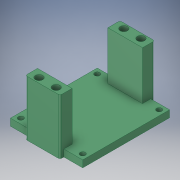
# Autodesk Inventor part: МД.001.1000 - Опора захвата
Saved by Autodesk Inventor 2019 (Build 230136000, 136)
## iProperties
Created: 2019-12-30
Part Number: МД.001.1000 - Опора захвата
Material: Пластик АБС
Document SubType Name: Modeling
Designer: Петров Иван
Density: 1.06 g/cm^3
Appearance: Гладкий — темный цвет морской волны
Author: Петров Иван
Autodesk Inventor part; units mm, degrees
ref_plane "YZ Plane" through (0, 0, 0) normal (1, 0, 0) x (0, 1, 0)
ref_plane "XZ Plane" through (0, 0, 0) normal (0, 1, 0) x (-1, 0, 0)
ref_plane "XY Plane" through (0, 0, 0) normal (0, 0, 1) x (1, 0, 0)
sketch "Эскиз1" plane through (0, 0, 0) normal (0, 1, 0) x (-1, 0, 0)
  circle A0 centre (38.8, 47.2) radius 1.5
  circle A1 centre (3, 47.2) radius 1.5
  circle A2 centre (38.8, 3) radius 1.5
  circle A3 centre (3, 3) radius 1.5
  line L0 (41.8, 0) -> (0, 0)
  line L1 (41.8, 0) -> (41.8, 50.2)
  line L2 (41.8, 50.2) -> (0, 50.2)
  line L3 (0, 0) -> (0, 50.2)
  point P0 (19.0194, 0)
  constraints: 8 end point, 4 centre point
extrude "Выдавливание1" add sketch "Эскиз1" along normal blind 4
sketch "Эскиз2" plane through (0, 4, 0) normal (0, 1, 0) x (1, 0, 0)
  line L0 (-41.8, -50.2) -> (0, -50.2) projected
  line L1 (-20.9, -50.2) -> (-20.9, -35.45)
  line L2 (-10.9, -45.45) -> (-30.9, -45.45)
  line L3 (-30.9, -45.45) -> (-30.9, -51.45)
  arc A0 (-30.9, -51.45) -> (-29.9, -52.45) centre (-29.9, -51.45) ccw
  line L4 (-29.9, -52.45) -> (-27.05, -52.45)
  line L5 (-27.05, -52.45) -> (-27.05, -51.384)
  arc A1 (-24.65, -51.384) -> (-27.05, -51.384) centre (-25.85, -49.6) ccw
  line L6 (-24.65, -51.384) -> (-24.65, -52.45)
  line L7 (-24.65, -52.45) -> (-17.15, -52.45)
  line L8 (-17.15, -52.45) -> (-17.15, -51.384)
  arc A2 (-14.75, -51.384) -> (-17.15, -51.384) centre (-15.95, -49.6) ccw
  line L9 (-14.75, -51.384) -> (-14.75, -52.45)
  line L10 (-14.75, -52.45) -> (-11.9, -52.45)
  arc A3 (-11.9, -52.45) -> (-10.9, -51.45) centre (-11.9, -51.45) ccw
  line L11 (-10.9, -51.45) -> (-10.9, -45.45)
  line L12 (-17.15, 2.25) -> (-17.15, 1.184)
  line L13 (-24.65, 2.25) -> (-17.15, 2.25)
  line L14 (-24.65, 1.184) -> (-24.65, 2.25)
  arc A4 (-27.05, 1.184) -> (-24.65, 1.184) centre (-25.85, -0.6) ccw
  line L15 (-27.05, 2.25) -> (-27.05, 1.184)
  line L16 (-29.9, 2.25) -> (-27.05, 2.25)
  arc A5 (-29.9, 2.25) -> (-30.9, 1.25) centre (-29.9, 1.25) ccw
  line L17 (-30.9, -4.75) -> (-30.9, 1.25)
  line L18 (-10.9, -4.75) -> (-30.9, -4.75)
  line L19 (-10.9, 1.25) -> (-10.9, -4.75)
  arc A6 (-10.9, 1.25) -> (-11.9, 2.25) centre (-11.9, 1.25) ccw
  line L20 (-14.75, 2.25) -> (-11.9, 2.25)
  line L21 (-14.75, 1.184) -> (-14.75, 2.25)
  arc A7 (-17.15, 1.184) -> (-14.75, 1.184) centre (-15.95, -0.6) ccw
  line L22 (-30.9, -45.45) -> (-30.9, -4.75)
  line L23 (-10.9, -4.75) -> (-10.9, -45.45)
  line L24 (-10.9, -45.45) -> (-30.9, -45.45)
  circle A8 centre (-20.9, -35.45) radius 1.25
  circle A9 centre (-20.9, -35.45) radius 3.4957
  circle A10 centre (-20.9, -35.45) radius 2.6787
  circle A11 centre (-20.9, -35.45) radius 5.4
  line L25 (-27.05, 2.25) -> (-24.65, 2.25)
  line L26 (-17.15, 2.25) -> (-14.75, 2.25)
  line L27 (-24.65, 2.25) -> (-21.4, 2.25)
  line L28 (-24.65, -52.45) -> (-17.15, -52.45)
  line L29 (-27.05, -52.45) -> (-24.65, -52.45)
  line L30 (-24.65, -52.45) -> (-17.15, -52.45)
  line L31 (-17.15, -52.45) -> (-14.75, -52.45)
  circle A12 centre (-25.85, -49.6) radius 2.15
  circle A13 centre (-15.95, -49.6) radius 2.15
  arc A14 (-17.15, 1.184) -> (-14.75, 1.184) centre (-15.95, -0.6) ccw
  circle A15 centre (-15.95, -0.6) radius 2.15
  circle A16 centre (-25.85, -0.6) radius 2.15
  point P0 (-10.9, -25.1)
  dimension "d2" = 14.75
  constraints: 62 end point, 18 point on circle, 16 centre point, 4 coincident, 4 collinear, 2 concentric, 1 midpoint, 1 vertical, 3 other
  measures "d2" distance of L1.start L1.end
extrude "Выдавливание2" add sketch "Эскиз2" against normal blind 4 and the other way blind 28 contours L3 L2 L1 L0 A1 | L0 A1 L5 L4 A0 L3 | A1 L0 | L0 A1 A12 | L0 A2 L8 L7 L6 A1 | A12 L6 L29 L5 | L2 L11 L0 A2 L1 | L17 A5 L16 L15 A4 L14 L13 L12 A7 L21 L20 A6 L19 L18 | A2 L0 | L0 A2 A13 | L11 A3 L10 L9 A2 L0 | A13 L9 L31 L8 | L25 L14 A16 L15 | A16 A4 | L21 A15 L12 L26 | A7 A15
sketch "Эскиз3" plane through (0, 32, 0) normal (0, 1, 0) x (1, 0, 0)
  line L0 (-41.8, -50.2) -> (0, -50.2)
  line L1 (-20.9, -50.2) -> (-20.9, -35.45)
  line L2 (-10.9, -45.45) -> (-30.9, -45.45)
  line L3 (-30.9, -45.45) -> (-30.9, -51.45)
  arc A0 (-30.9, -51.45) -> (-29.9, -52.45) centre (-29.9, -51.45) ccw
  line L4 (-29.9, -52.45) -> (-27.05, -52.45)
  line L5 (-27.05, -52.45) -> (-27.05, -51.384)
  arc A1 (-24.65, -51.384) -> (-27.05, -51.384) centre (-25.85, -49.6) ccw
  line L6 (-24.65, -51.384) -> (-24.65, -52.45)
  line L7 (-24.65, -52.45) -> (-17.15, -52.45)
  line L8 (-17.15, -52.45) -> (-17.15, -51.384)
  arc A2 (-14.75, -51.384) -> (-17.15, -51.384) centre (-15.95, -49.6) ccw
  line L9 (-14.75, -51.384) -> (-14.75, -52.45)
  line L10 (-14.75, -52.45) -> (-11.9, -52.45)
  arc A3 (-11.9, -52.45) -> (-10.9, -51.45) centre (-11.9, -51.45) ccw
  line L11 (-10.9, -51.45) -> (-10.9, -45.45)
  line L12 (-17.15, 2.25) -> (-17.15, 1.184)
  line L13 (-24.65, 2.25) -> (-17.15, 2.25)
  line L14 (-24.65, 1.184) -> (-24.65, 2.25)
  arc A4 (-27.05, 1.184) -> (-24.65, 1.184) centre (-25.85, -0.6) ccw
  line L15 (-27.05, 2.25) -> (-27.05, 1.184)
  line L16 (-29.9, 2.25) -> (-27.05, 2.25)
  arc A5 (-29.9, 2.25) -> (-30.9, 1.25) centre (-29.9, 1.25) ccw
  line L17 (-30.9, -4.75) -> (-30.9, 1.25)
  line L18 (-10.9, -4.75) -> (-30.9, -4.75)
  line L19 (-10.9, 1.25) -> (-10.9, -4.75)
  arc A6 (-10.9, 1.25) -> (-11.9, 2.25) centre (-11.9, 1.25) ccw
  line L20 (-14.75, 2.25) -> (-11.9, 2.25)
  line L21 (-14.75, 1.184) -> (-14.75, 2.25)
  arc A7 (-17.15, 1.184) -> (-14.75, 1.184) centre (-15.95, -0.6) ccw
  line L22 (-30.9, -45.45) -> (-30.9, -4.75)
  line L23 (-10.9, -4.75) -> (-10.9, -45.45)
  line L24 (-10.9, -45.45) -> (-30.9, -45.45)
  circle A8 centre (-20.9, -35.45) radius 1.25
  circle A9 centre (-20.9, -35.45) radius 3.4957
  circle A10 centre (-20.9, -35.45) radius 2.6787
  circle A11 centre (-20.9, -35.45) radius 5.4
  line L25 (-27.05, 2.25) -> (-24.65, 2.25)
  line L26 (-17.15, 2.25) -> (-14.75, 2.25)
  line L27 (-24.65, 2.25) -> (-21.4, 2.25)
  line L28 (-24.65, -52.45) -> (-17.15, -52.45)
  line L29 (-27.05, -52.45) -> (-24.65, -52.45)
  line L30 (-24.65, -52.45) -> (-17.15, -52.45)
  line L31 (-17.15, -52.45) -> (-14.75, -52.45)
  circle A12 centre (-25.85, -49.6) radius 2.15
  circle A13 centre (-15.95, -49.6) radius 2.15
  arc A14 (-17.15, 1.184) -> (-14.75, 1.184) centre (-15.95, -0.6) ccw
  circle A15 centre (-15.95, -0.6) radius 2.15
  circle A16 centre (-25.85, -0.6) radius 2.15
  point P0 (0, 0)
  point P1 (-10.9, -25.1)
  dimension "d7" = 14.75
  constraints: 64 end point, 18 point on circle, 16 centre point, 4 coincident, 4 collinear, 2 concentric, 1 midpoint, 1 vertical, 3 other
  measures "d7" distance of L1.start L1.end
extrude "Выдавливание3" cut sketch "Эскиз3" against normal blind 10 contours A1 L0 | L0 A1 A12 | A2 L0 | L0 A2 A13 | A16 A4 | A7 A15
